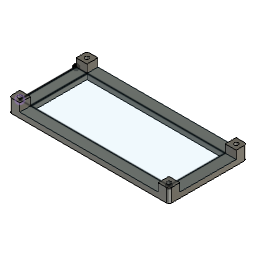
PicoDebuggerMount (Autodesk Fusion 360 design; units mm, degrees)
Autodesk Fusion 360 part; units mm, degrees
sketch "Base and Mounts" plane through (0, 0, 0) normal (0, 0, 1) x (1, 0, 0)
  line L0 (-55.5, 25) -> (55.5, 25) construction
  line L1 (55.5, 25) -> (55.5, -25) construction
  line L2 (55.5, -25) -> (-55.5, -25) construction
  line L3 (-55.5, -25) -> (-55.5, 25) construction
  line L4 (-55.5, 25) -> (55.5, -25) construction
  line L5 (55.5, 25) -> (-55.5, -25) construction
  circle A0 centre (-55.5, 25) radius 1.55
  circle A1 centre (55.5, 25) radius 1.55
  circle A2 centre (-55.5, -25) radius 1.55
  circle A3 centre (55.5, -25) radius 1.55
  line L6 (-59.55, 29.05) -> (-51.45, 29.05)
  line L7 (-51.45, 29.05) -> (-51.45, 20.95)
  line L8 (-51.45, 20.95) -> (-59.55, 20.95)
  line L9 (-59.55, 20.95) -> (-59.55, 29.05)
  line L10 (-59.55, 29.05) -> (-51.45, 20.95) construction
  line L11 (-51.45, 29.05) -> (-59.55, 20.95) construction
  line L12 (51.45, 29.05) -> (59.55, 29.05)
  line L13 (59.55, 29.05) -> (59.55, 20.95)
  line L14 (59.55, 20.95) -> (51.45, 20.95)
  line L15 (51.45, 20.95) -> (51.45, 29.05)
  line L16 (51.45, 29.05) -> (59.55, 20.95) construction
  line L17 (59.55, 29.05) -> (51.45, 20.95) construction
  line L18 (51.45, -20.95) -> (59.55, -20.95)
  line L19 (59.55, -20.95) -> (59.55, -29.05)
  line L20 (59.55, -29.05) -> (51.45, -29.05)
  line L21 (51.45, -29.05) -> (51.45, -20.95)
  line L22 (51.45, -20.95) -> (59.55, -29.05) construction
  line L23 (59.55, -20.95) -> (51.45, -29.05) construction
  line L24 (-59.55, -20.95) -> (-51.45, -20.95)
  line L25 (-51.45, -20.95) -> (-51.45, -29.05)
  line L26 (-51.45, -29.05) -> (-59.55, -29.05)
  line L27 (-59.55, -29.05) -> (-59.55, -20.95)
  line L28 (-59.55, -20.95) -> (-51.45, -29.05) construction
  line L29 (-51.45, -20.95) -> (-59.55, -29.05) construction
  line L30 (-51.45, 29.05) -> (51.45, 29.05)
  line L31 (59.55, 20.95) -> (59.55, -20.95)
  line L32 (51.45, -29.05) -> (-51.45, -29.05)
  line L33 (-59.55, -20.95) -> (-59.55, 20.95)
  point P0 (-55.5, 25)
  point P1 (55.5, 25)
  point P2 (55.5, -25)
  point P3 (-55.5, -25)
  dimension "d6" = 111
  dimension "d7" = 50
  dimension "d8" = 3.1
  dimension "d9" = 3.1
  dimension "d10" = 3.1
  dimension "d11" = 3.1
  dimension "d12" = 4.05
  dimension "d13" = 4.05
  dimension "d14" = 4.05
  dimension "d15" = 4.05
  dimension "d16" = 4.05
  dimension "d17" = 4.05
  dimension "d18" = 4.05
  dimension "d19" = 4.05
  dimension "d25" = 4.05
  constraint horizontal L0
  constraint perpendicular L0 L1
  constraint parallel L0 L2
  constraint parallel L1 L3
  constraint coincident L4 origin
  constraint coincident L5 origin
  constraint coincident P0 L0.start
  constraint coincident P1 L0.end
  constraint coincident P3 L2.end
  constraint coincident P2 L1.end
  constraint horizontal L6
  constraint perpendicular L6 L7
  constraint parallel L6 L8
  constraint parallel L7 L9
  constraint coincident L10 P0
  constraint coincident L11 P0
  constraint horizontal L12
  constraint perpendicular L12 L13
  constraint parallel L12 L14
  constraint parallel L13 L15
  constraint coincident L16 P1
  constraint coincident L17 P1
  constraint horizontal L18
  constraint perpendicular L18 L19
  constraint parallel L18 L20
  constraint parallel L19 L21
  constraint coincident L22 P2
  constraint coincident L23 P2
  constraint horizontal L24
  constraint perpendicular L24 L25
  constraint parallel L24 L26
  constraint parallel L25 L27
  constraint coincident L28 P3
  constraint coincident L29 P3
  constraint coincident L2 P3
  measures "d6" distance of P2 L2.end
  measures "d7" distance of P1 L1.end
  measures "d8" diameter of A0
  measures "d9" diameter of A1
  measures "d10" diameter of A2
  measures "d11" diameter of A3
  measures "d12" distance of P0 L7
  measures "d13" distance of P0 L6
  measures "d14" distance of P1 L12
  measures "d15" distance of P1 L13
  measures "d16" distance of P2 L19
  measures "d17" distance of P2 L20
  measures "d18" distance of P3 L24
  measures "d19" distance of P3 L25
  measures "d25" distance of P3 L27
extrude "Extrude1" add sketch "Base and Mounts" along normal blind 10 contours L6 L7 L8 L9 | L12 L13 L14 L15 | L24 L25 L26 L27 | L18 L19 L20 L21 makes body 1 at (56.7356, 25.9359, 6.6667) makes body 2 at (55.4614, -23.4505, 6.6667) makes body 3 at (-55.5386, 26.5495, 6.6667) makes body 4 at (-54.2644, -24.0641, 6.6667)
extrude "Extrude2" add sketch "Base and Mounts" along normal blind 4 contours L7 L8 L14 L15 L18 L21 L24 L25 L30 L31 L32 L33 bodies 1 2 3 4
sketch "Cutouts" plane through (0, 0, 4) normal (0, 0, 1) x (-1, 0, 0)
  line L0 (51.45, 20.95) -> (51.45, 29.05)
  line L1 (51.45, 29.05) -> (-51.45, 29.05)
  line L2 (-51.45, 29.05) -> (-51.45, 20.95)
  line L3 (-51.45, 20.95) -> (-59.55, 20.95)
  line L4 (-59.55, 20.95) -> (-59.55, -20.95)
  line L5 (-59.55, -20.95) -> (-51.45, -20.95)
  line L6 (-51.45, -20.95) -> (-51.45, -29.05)
  line L7 (-51.45, -29.05) -> (51.45, -29.05)
  line L8 (51.45, -29.05) -> (51.45, -20.95)
  line L9 (51.45, -20.95) -> (59.55, -20.95)
  line L10 (59.55, -20.95) -> (59.55, 20.95)
  line L11 (59.55, 20.95) -> (51.45, 20.95)
  line L12 (59.55, -20.95) -> (59.549, -20.95)
  line L13 (59.549, -20.95) -> (59.549, 20.95)
  line L14 (59.549, 20.95) -> (59.55, 20.95)
  line L15 (59.55, 20.95) -> (59.55, -20.95)
  line L16 (59.549, -20.95) -> (51.449, -20.95)
  line L17 (51.449, -20.95) -> (51.449, 20.95)
  line L18 (51.449, 20.95) -> (59.549, 20.95)
  line L19 (59.549, 20.95) -> (59.549, -20.95)
  line L20 (51.449, -20.95) -> (-51.45, -20.95)
  line L21 (-51.45, -20.95) -> (-51.45, 20.95)
  line L22 (-51.45, 20.95) -> (51.449, 20.95)
  line L23 (51.449, 20.95) -> (51.449, -20.95)
  point P0 (59.55, 20.95)
  dimension "d27" = 0.001
  dimension "d28" = 8.1
  dimension "d29" = 41.9
  dimension "d30" = 8.101
  dimension "d41" = 41.9
  dimension "d42" = 41.9
  constraint horizontal L12
  constraint vertical L13
  constraint horizontal L14
  constraint vertical L15
  constraint coincident L9.end L10.start
  constraint horizontal L16
  constraint vertical L17
  constraint horizontal L18
  constraint vertical L19
  constraint horizontal L20
  constraint vertical L21
  constraint horizontal L22
  constraint vertical L23
  constraint coincident L2.end L3.start
  measures "d27" distance of L13.end P0
  measures "d28" distance of L17.end L13.end
  measures "d29" distance of L16.end L17.end
  measures "d30" distance of L17 P0
  measures "d41" distance of L9.end P0
  measures "d42" distance of L9.end P0
extrude "Extrude3" cut sketch "Cutouts" against normal up to surface (4 mm away) contours L17 L20 L21 L22 L23 bodies 1
extrude "Extrude4" cut sketch "Cutouts" against normal up to surface (4 mm away) contours L9 L10 L11 L12 L13 L14 L15 L19 bodies 1
fillet "Fillet5" radius 2 4 edges at (59.55, -29.05, 5) (-59.55, -29.05, 5) (-59.55, 29.05, 5) (59.55, 29.05, 5) on bodies 1
equation "HoleSpacingX = 50 mm"
equation "HoleSpacingY = 111 mm"
equation "ThreadedInsertDiameter = 3.1 mm"
equation "ThreadedInsertHeight = 4 mm"
equation "ThreadedInsertClearance = 2.5 mm"
equation "d6 = HoleSpacingY"
equation "d7 = HoleSpacingX"
equation "d8 = ThreadedInsertDiameter"
equation "d9 = ThreadedInsertDiameter"
equation "d10 = ThreadedInsertDiameter"
equation "d11 = ThreadedInsertDiameter"
equation "d12 = ThreadedInsertClearance + ( ThreadedInsertDiameter / 2 )"
equation "d13 = d12"
equation "d14 = d12"
equation "d15 = d12"
equation "d16 = d12"
equation "d17 = d12"
equation "d18 = d12"
equation "d19 = d12"
equation "MountHeight = 6 mm"
equation "d21 = MountHeight + ThreadedInsertHeight"
equation "d23 = ThreadedInsertHeight"
equation "d25 = d12"
equation "DebugHeaderCutoutWidth = 0.001 mm"
equation "d27 = DebugHeaderCutoutWidth"
equation "d28 = 2 * d12"
equation "d29 = d42"
equation "d41 = d42"
named bodies: "Base and Mounts"
